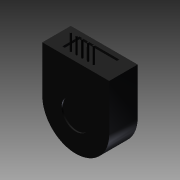
# Autodesk Inventor part: USD S1-100-B Housing
Saved by Autodesk Inventor 2012 (Build 160160000, 160)
## iProperties
Created: 2012-07-07
Part Number: USD S1-100-B Housing
Material: Default
Document SubType Name: Modeling
Designer: Programming Team
Density: 1 g/cm^3
Author: Programming Team
Autodesk Inventor part; units mm, degrees
ref_plane "YZ Plane" through (0, 0, 0) normal (1, 0, 0) x (0, 1, 0)
ref_plane "XZ Plane" through (0, 0, 0) normal (0, 1, 0) x (-1, 0, 0)
ref_plane "XY Plane" through (0, 0, 0) normal (0, 0, 1) x (1, 0, 0)
sketch "Sketch1" plane through (0, 0, 0) normal (0, 0, 1) x (1, 0, 0)
  arc A0 (-14.9225, 0) -> (14.9225, 0) centre (0, 0) ccw
  line L0 (-14.9225, 0) -> (-14.9225, 20.6375)
  line L1 (-14.9225, 20.6375) -> (14.9225, 20.6375)
  line L2 (14.9225, 20.6375) -> (14.9225, 0)
  circle A1 centre (0, 0) radius 4.6736
  circle A2 centre (0, 0) radius 3.175
  line L3 (14.9225, 0) -> (14.9225, -0.9265)
  circle A3 centre (0, 0) radius 6.35
  dimension "d0" = 29.845
  dimension "d2" = 9.3472
  dimension "d3" = 6.35
  dimension "d6" = 12.7
  dimension "d24" = 35.56
  constraints: 8 end point, 4 centre point, 4 coincident, 3 tangent, 2 parallel, 2 point on circle, 1 perpendicular, 1 vertical
  measures "d0" diameter of A0
  measures "d2" diameter of A1
  measures "d3" diameter of A2
  measures "d6" diameter of A3
extrude "Extrusion2" add sketch "Sketch1" against normal blind 12.7 contours L0 L1 L2 A0 | A1 | A2 | A3
extrude "Extrusion3" cut sketch "Sketch1" against normal blind 0.6096 contours A1 | A2 | A3
sketch "Sketch2" plane through (-14.9225, 20.6375, 0) normal (0, 1, 0) x (1, 0, 0)
  line L0 (0, 0) -> (0, 12.7) projected
  line L1 (29.845, 0) -> (0, 0) projected
  line L2 (29.845, 0) -> (29.845, 12.7) projected
  line L3 (6.0325, 10.541) -> (23.8125, 10.541)
  line L4 (23.8125, 10.541) -> (23.8125, 2.921)
  line L5 (23.8125, 2.921) -> (6.0325, 2.921)
  line L6 (6.0325, 2.921) -> (6.0325, 10.541)
  circle A0 centre (9.8425, 2.921) radius 0.381
  circle A1 centre (12.3825, 2.921) radius 0.381
  circle A2 centre (14.9225, 2.921) radius 0.381
  circle A3 centre (17.4625, 2.921) radius 0.381
  circle A4 centre (20.0025, 2.921) radius 0.381
  point P0 (14.9225, 0)
  dimension "d11" = 17.78
  dimension "d12" = 8.89
  dimension "d13" = 7.62
  dimension "d14" = 2.921
  dimension "d15" = 0.762
  dimension "d16" = 9.8425
  dimension "d19" = 2.54
  dimension "d25" = 9.8425
  constraints: 8 end point, 5 centre point, 2 horizontal, 2 parallel, 1 perpendicular, 1 point on line, 8 other
  measures "d11" distance of L3.start L3.end
  measures "d12" distance from line of point (14.923, 0) L6
  measures "d13" distance of L3.end L4.end
  measures "d14" distance between parallel lines of L1 L5
  measures "d15" diameter of A0
  measures "d16" distance from line of L0 A0.centre
  measures "d19" distance of A0.centre A1.centre
  measures "d25" distance from line of L2 A4.centre
extrude "Extrusion4" cut sketch "Sketch2" against normal blind 1.0668 contours L3 L4 L5 A4 A3 A2 A1 A0 L6 | A0 L5 | L5 A4 | A1 L5 | L5 A3 | A2 L5 picked at (9.9376, 3.0052) picked at (19.9292, 3.1544) picked at (12.4776, 3.0052) picked at (17.3892, 3.1544) picked at (15.0176, 3.0052)
extrude "Extrusion5" add sketch "Sketch2" along normal blind 7.3152 contours A0 L5 | L5 A0 | A4 L5 | L5 A4 | A1 L5 | L5 A1 | A3 L5 | L5 A3 | A2 L5 | L5 A2
equation "\"d12\" = 0.5 * d11"
body "Solid2"
